PLATE_HV_BOTTOM (Autodesk Fusion 360 design; units mm, degrees)
Autodesk Fusion 360 part; units mm, degrees
note: some values were not read from the file. Set by a fixed rule: which sketch regions a step uses.
sketch "Esquisse1" plane through (0, 0, 0) normal (0, 0, 1) x (1, 0, 0)
  line L0 (100, 78) -> (-100, 78)
  line L1 (-100, 78) -> (-100, -78)
  line L2 (-100, -78) -> (100, -78)
  line L3 (100, -78) -> (100, 78)
  line L4 (100, 78) -> (-100, -78) construction
  line L5 (-100, 78) -> (100, -78) construction
  line L6 (103, -75) -> (-103, -75)
  line L7 (-103, -75) -> (-103, 75)
  line L8 (-103, 75) -> (103, 75)
  line L9 (103, 75) -> (103, -75)
  line L10 (103, -75) -> (-103, 75) construction
  line L11 (-103, -75) -> (103, 75) construction
  dimension "d1" = 200
  dimension "d2" = 206
  dimension "d3" = 150
  dimension "d4" = 156
  constraint horizontal L0
  constraint perpendicular L0 L1
  constraint parallel L0 L2
  constraint parallel L1 L3
  constraint coincident L4 origin
  constraint coincident L5 origin
  constraint horizontal L6
  constraint perpendicular L6 L7
  constraint parallel L6 L8
  constraint parallel L7 L9
  constraint coincident L10 origin
  constraint coincident L11 origin
  measures "d1" distance of L0.start L0.end
  measures "d2" distance of L7.end L8.end
  measures "d3" distance of L6.end L7.end
  measures "d4" distance of L0.end L1.end
extrude "Extrusion1" add sketch "Esquisse1" along normal blind 3
sketch "Esquisse7" plane through (0, 0, 3) normal (0, 0, 1) x (-1, 0, 0)
  line L0 (-100, 78) -> (-100, 75)
  line L1 (-100, -75) -> (-100, -78)
  line L2 (-100, -78) -> (100, -78)
  line L3 (100, -78) -> (100, -75)
  line L4 (100, 75) -> (100, 78)
  line L5 (100, 78) -> (-100, 78)
  line L6 (34.35, -19.5) -> (38.35, -19.5)
  line L7 (34.35, -17.9) -> (34.35, -19.5)
  line L8 (38.35, -17.9) -> (34.35, -17.9)
  line L9 (38.35, -19.5) -> (38.35, -17.9)
  line L10 (38.35, 19.5) -> (38.35, 17.9)
  line L11 (38.35, 17.9) -> (34.35, 17.9)
  line L12 (34.35, 19.5) -> (38.35, 19.5)
  line L13 (34.35, 17.9) -> (34.35, 19.5)
  line L14 (53.45, -17.9) -> (53.45, -19.5)
  line L15 (53.45, -19.5) -> (49.45, -19.5)
  line L16 (49.45, -17.9) -> (53.45, -17.9)
  line L17 (49.45, -19.5) -> (49.45, -17.9)
  line L18 (53.45, 19.5) -> (53.45, 17.9)
  line L19 (49.45, 17.9) -> (49.45, 19.5)
  line L20 (49.45, 19.5) -> (53.45, 19.5)
  line L21 (53.45, 17.9) -> (49.45, 17.9)
  line L22 (34.35, -17.9) -> (38.35, -17.9)
  line L23 (38.35, -19.5) -> (34.35, -19.5)
  line L24 (34.35, -19.5) -> (34.35, -17.9)
  line L25 (38.35, -17.9) -> (38.35, -19.5)
  circle A0 centre (-34.35, -6.2) radius 1.8
  circle A1 centre (-34.35, 10.5) radius 1.8
  line L26 (100, -75) -> (103, -75)
  line L27 (103, -75) -> (103, 75)
  line L28 (103, 75) -> (100, 75)
  line L29 (-100, 75) -> (-103, 75)
  line L30 (-103, 75) -> (-103, -75)
  line L31 (-103, -75) -> (-100, -75)
  dimension "d87" = 1.6
  dimension "d88" = 4
  dimension "d89" = 1.6
  dimension "d90" = 4
  dimension "d91" = 4
  dimension "d92" = 1.6
  dimension "d93" = 4
  dimension "d94" = 1.6
  dimension "d95" = 3.6
  dimension "d96" = 3.6
  dimension "d97" = 16.7
  dimension "d98" = 35.8
  dimension "d99" = 11.1
  dimension "d100" = 35.8
  dimension "d101" = 35.8
  dimension "d102" = 11.1
  dimension "d103" = 37.4813
  dimension "d114" = 68.7
  dimension "d115" = 11.7
  dimension "d116" = 68.7
  dimension "d118" = 17.9
  dimension "d119" = 34.35
  dimension "d141" = 9
  constraint parallel L20 L21
  constraint parallel L11 L12
  constraint parallel L15 L16
  constraint parallel L6 L8
  constraint parallel L9 L24
  constraint parallel L14 L17
  constraint parallel L18 L19
  constraint parallel L10 L13
  constraint parallel L16 L21
  constraint parallel L8 L11
  constraint parallel L9 L17
  constraint parallel L10 L19
  constraint perpendicular L18 L20
  constraint perpendicular L10 L12
  constraint perpendicular L14 L16
  measures "d87" distance of L18.start L18.end
  measures "d88" distance of L18.start L19.end
  measures "d89" distance of L14.start L14.end
  measures "d90" distance of L14.end L15.end
  measures "d91" distance of L6.start L6.end
  measures "d92" distance of L6.end L8.start
  measures "d93" distance of L10.end L11.end
  measures "d94" distance of L10.start L10.end
  measures "d95" diameter of A1
  measures "d96" diameter of A0
  measures "d97" distance of A0.centre A1.centre
  measures "d98" distance of L8 L11
  measures "d99" distance of L10 L19
  measures "d100" distance of L16 L21
  measures "d101" distance of L21 L22
  measures "d102" distance of L9 L17
  measures "d103" distance of L8.start L19.start
  measures "d114" horizontal distance of L7.start A0.centre
  measures "d115" vertical distance of L7.start A0.centre
  measures "d116" horizontal distance of L11.end A1.centre
  measures "d118" vertical distance of origin L7.start
  measures "d119" horizontal distance of origin L7.start
  measures "d141" distance of L12 A1.centre
extrude "Extrusion4" cut sketch "Esquisse7" against normal blind 3 contours L6 L7 L8 L9 L22 L23 L24 L25 | L10 L11 L12 L13 | L14 L15 L16 L17 | L18 L19 L20 L21 | A0 | A1
sketch "Esquisse9" plane through (0, 0, 0) normal (0, 0, -1) x (1, 0, 0)
  line L0 (-100, -78) -> (100, -78)
  line L1 (100, -78) -> (100, -75)
  line L2 (100, 75) -> (100, 78)
  line L3 (100, 78) -> (-100, 78)
  line L4 (-100, 78) -> (-100, 75)
  line L5 (-100, -75) -> (-100, -78)
  line L6 (100, -75) -> (103, -75)
  line L7 (103, -75) -> (103, 75)
  line L8 (103, 75) -> (100, 75)
  line L9 (-100, 75) -> (-103, 75)
  line L10 (-103, 75) -> (-103, -75)
  line L11 (-103, -75) -> (-100, -75)
  line L12 (-34.35, -17.9) -> (-34.35, -19.5)
  line L13 (-34.35, -19.5) -> (-38.35, -19.5)
  line L14 (-38.35, -19.5) -> (-38.35, -17.9)
  line L15 (-38.35, -17.9) -> (-34.35, -17.9)
  line L16 (-53.45, 19.5) -> (-49.45, 19.5)
  line L17 (-49.45, 19.5) -> (-49.45, 17.9)
  line L18 (-49.45, 17.9) -> (-53.45, 17.9)
  line L19 (-53.45, 17.9) -> (-53.45, 19.5)
  circle A0 centre (34.35, 10.5) radius 1.8
  line L20 (-53.45, -19.5) -> (-53.45, -17.9)
  line L21 (-53.45, -17.9) -> (-49.45, -17.9)
  line L22 (-49.45, -17.9) -> (-49.45, -19.5)
  line L23 (-49.45, -19.5) -> (-53.45, -19.5)
  line L24 (-38.35, 17.9) -> (-38.35, 19.5)
  line L25 (-38.35, 19.5) -> (-34.35, 19.5)
  line L26 (-34.35, 19.5) -> (-34.35, 17.9)
  line L27 (-34.35, 17.9) -> (-38.35, 17.9)
  circle A1 centre (34.35, -6.2) radius 1.8
sketch "Esquisse10" plane through (0, 0, 3) normal (0, 0, 1) x (-1, 0, 0)
  line L0 (34.35, -19.5) -> (34.35, -17.9)
  line L1 (34.35, -17.9) -> (38.35, -17.9)
  line L2 (38.35, -17.9) -> (38.35, -19.5)
  line L3 (38.35, -19.5) -> (34.35, -19.5)
  line L4 (49.45, 19.5) -> (53.45, 19.5)
  line L5 (53.45, 19.5) -> (53.45, 17.9)
  line L6 (53.45, 17.9) -> (49.45, 17.9)
  line L7 (49.45, 17.9) -> (49.45, 19.5)
  line L8 (53.45, -17.9) -> (53.45, -19.5)
  line L9 (53.45, -19.5) -> (49.45, -19.5)
  line L10 (49.45, -19.5) -> (49.45, -17.9)
  line L11 (49.45, -17.9) -> (53.45, -17.9)
  line L12 (38.35, 19.5) -> (38.35, 17.9)
  line L13 (38.35, 17.9) -> (34.35, 17.9)
  line L14 (34.35, 17.9) -> (34.35, 19.5)
  line L15 (34.35, 19.5) -> (38.35, 19.5)
  line L16 (-100, -75) -> (-100, -78)
  line L17 (-100, -78) -> (100, -78)
  line L18 (100, -78) -> (100, -75)
  line L19 (100, -75) -> (103, -75)
  line L20 (103, -75) -> (103, 75)
  line L21 (103, 75) -> (100, 75)
  line L22 (100, 75) -> (100, 78)
  line L23 (100, 78) -> (-100, 78)
  line L24 (-100, 78) -> (-100, 75)
  line L25 (-100, 75) -> (-103, 75)
  line L26 (-103, 75) -> (-103, -75)
  line L27 (-103, -75) -> (-100, -75)
  line L28 (68, 20) -> (78, 20)
  line L29 (83, 15) -> (83, -15)
  line L30 (78, -20) -> (68, -20)
  line L31 (63, -15) -> (63, 15)
  line L32 (63, 20) -> (83, -20) construction
  line L33 (83, 20) -> (63, -20) construction
  arc A0 (78, -20) -> (83, -15) centre (78, -15) ccw
  arc A1 (63, -15) -> (68, -20) centre (68, -15) ccw
  arc A2 (68, 20) -> (63, 15) centre (68, 15) ccw
  arc A3 (83, 15) -> (78, 20) centre (78, 15) ccw
  point P0 (73, 0)
  dimension "d134" = 5
  dimension "d142" = 20
  dimension "d143" = 40
  dimension "d144" = 20
  constraint horizontal L28
  constraint perpendicular L28 L29
  constraint parallel L28 L30
  constraint parallel L29 L31
  constraint coincident L32 P0
  constraint coincident L33 P0
  constraint coincident L32.end L29
  constraint coincident L32.end L30
  constraint tangent L29 A0
  constraint tangent L30 A0
  constraint coincident L33.end L31
  constraint coincident L33.end L30
  constraint tangent L31 A1
  constraint tangent L30 A1
  constraint equal A0 A1
  constraint coincident L32.start L31
  constraint coincident L32.start L28
  constraint tangent L31 A2
  constraint tangent L28 A2
  constraint equal A0 A2
  constraint coincident L33.start L28
  constraint coincident L33.start L29
  constraint tangent L28 A3
  constraint tangent L29 A3
  constraint equal A0 A3
  measures "d134" radius of A0
  measures "d142" distance of L20 L29
  measures "d143" distance of L28 L30
  measures "d144" distance of L29 L31
extrude "Extrusion6" cut sketch "Esquisse10" against normal blind 3 contours L28 L29 L30 L31 A0 A1 A2 A3
equation "Transfo_notch_larg_Ref = 1.6 mm" comment "epaisseur des encoches du transfo"
equation "Trasnfo_notch_long_Ref = 4 mm" comment "Longueurs des encoches du transfo"
equation "Transfo_Dist_Larg_2_notchs_Ref = 11.9 mm" comment "Distance entre deux encoches (largeur)"
equation "Transfo_Dist_Long_2_nothcs_Ref = 39 mm - ( 2 * 1.6 ) * 1 mm" comment "Distance (longueur) entre deux encoches"
equation "Transfo_Hole_Diam_Ref = 3.7 mm" comment "Diamètre des trous du transfo"
equation "Transfo_Dist_2_Hole_Ref = 16.7 mm" comment "Distance entre les centres des trous du transfo"
equation "Transfo_Dist_Notch_Hole_Ref = 69.2 mm" comment "Distance (minimal) entre les encoches et les trous"
equation "d115 = d98 - d97 - d141 + d87"
equation "d118 = d98 / 2"
equation "d119 = d114 / 2"
